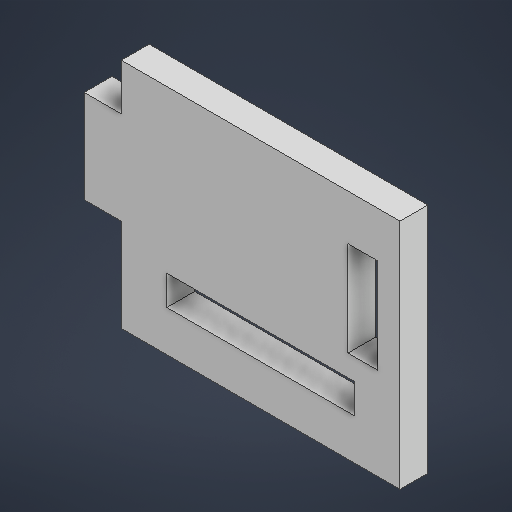
# Autodesk Inventor part: Battary_holder
Saved by Autodesk Inventor 2027 (Build 310192000, 192)
## iProperties
Created: 2026-05-15
Part Number: Battary_holder
Material: Generic
Document SubType Name: Modeling
Designer: alexy
Density: 1 g/cm^3
Appearance: Default
Author: alexy
Autodesk Inventor part; units mm, degrees
ref_plane "YZ Plane" through (0, 0, 0) normal (1, 0, 0) x (0, 1, 0)
ref_plane "XZ Plane" through (0, 0, 0) normal (0, 1, 0) x (-1, 0, 0)
ref_plane "XY Plane" through (0, 0, 0) normal (0, 0, 1) x (1, 0, 0)
sketch "Sketch1" plane through (0, 0, 0) normal (0, 0, 1) x (1, 0, 0)
  line L0 (0, 10) -> (-4, 10)
  line L1 (-4, 10) -> (-4, 20)
  line L2 (-4, 20) -> (0, 20)
  line L3 (0, 20) -> (0, 10)
  line L4 (0, 10) -> (0, 0)
  line L5 (0, 0) -> (30, 0)
  line L6 (30, 0) -> (30, 25)
  line L7 (30, 25) -> (0, 25)
  line L8 (0, 25) -> (0, 20)
  line L9 (4.9, 7.6) -> (25.1, 7.6)
  line L10 (25.1, 7.6) -> (25.1, 4.4)
  line L11 (25.1, 4.4) -> (4.9, 4.4)
  line L12 (4.9, 4.4) -> (4.9, 7.6)
  line L13 (4.9, 7.6) -> (25.1, 4.4) construction
  line L14 (25.1, 7.6) -> (4.9, 4.4) construction
  line L15 (24.4, 20.1) -> (27.6, 20.1)
  line L16 (27.6, 20.1) -> (27.6, 9.9)
  line L17 (27.6, 9.9) -> (24.4, 9.9)
  line L18 (24.4, 9.9) -> (24.4, 20.1)
  line L19 (24.4, 20.1) -> (27.6, 9.9) construction
  line L20 (27.6, 20.1) -> (24.4, 9.9) construction
  point P0 (15, 6)
  point P1 (15, 0)
  point P2 (26, 15)
  point P3 (0, 15)
  dimension "d0" = 10
  dimension "d1" = 4
  dimension "d3" = 10
  dimension "d4" = 30
  dimension "d5" = 20.2
  dimension "d6" = 3.2
  dimension "d7" = 5
  dimension "d8" = 6
  dimension "d11" = 3.2
  dimension "d12" = 4
  dimension "d13" = 10.2
  constraints: 42 end point, 7 perpendicular, 6 midpoint, 6 parallel, 3 horizontal, 2 vertical alignment, 1 horizontal alignment, 1 point on line, 1 vertical
  measures "d0" distance of L0.end L1.end
  measures "d1" distance of L1.end L2.end
  measures "d3" distance from line of L4.end L0
  measures "d4" distance of L4.end L5.end
  measures "d5" distance of L10.end L11.end
  measures "d6" distance of L9.end L10.end
  measures "d7" distance of L7.end L2.end
  measures "d8" vertical distance of L4.end point (15, 6)
  measures "d11" distance of L15.start L15.end
  measures "d12" distance from line of L6 point (26, 15)
  measures "d13" distance of L15.end L16.end
extrude "Extrusion1" add sketch "Sketch1" along normal blind 3
body "Solid1"
